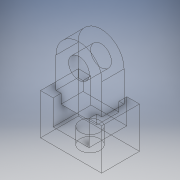
# Autodesk Inventor part: connectiong-rod-star-side
Saved by Autodesk Inventor 2018 (Build 220112000, 112)
## iProperties
Created: 2025-07-17
Part Number: connectiong-rod-star-side
Material: Generic
Document SubType Name: Modeling
Designer: neo
Density: 1 g/cm^3
Appearance: Default
Author: neo
Autodesk Inventor part; units mm, degrees
ref_plane "YZ Plane" through (0, 0, 0) normal (1, 0, 0) x (0, 1, 0)
ref_plane "XZ Plane" through (0, 0, 0) normal (0, 1, 0) x (-1, 0, 0)
ref_plane "XY Plane" through (0, 0, 0) normal (0, 0, 1) x (1, 0, 0)
sketch "Sketch1" plane through (0, 0, 0) normal (0, 1, 0) x (-1, 0, 0)
  circle A0 centre (0, 0) radius 1.65
  arc A1 (3.65, 0) -> (-3.65, 0) centre (0, 0) ccw
  line L0 (-3.65, 0) -> (-3.65, -11.35)
  line L1 (-3.65, -11.35) -> (3.65, -11.35)
  line L2 (3.65, -11.35) -> (3.65, 0)
  line L3 (0, 0) -> (0, -26.2529)
  line L4 (2.85, -11.35) -> (-2.85, -11.35)
  line L5 (-2.85, -9.35) -> (-2.85, -6.35)
  line L6 (-2.85, -6.35) -> (2.85, -6.35)
  line L7 (2.85, -6.35) -> (2.85, -9.35)
  line L8 (2.85, -9.35) -> (-2.85, -9.35)
  dimension "d0" = 3.3
  dimension "d1" = 2
  dimension "d2" = 15
  dimension "d3" = 5.7
  dimension "d4" = 5
  dimension "d5" = 2
  dimension "d13" = 3.65
  dimension "d14" = 7.3
  dimension "d15" = 0.8
  constraints: 18 end point, 3 parallel, 2 centre point, 2 coincident, 2 perpendicular, 2 point on circle, 2 tangent, 1 horizontal, 1 point on line, 1 vertical, 1 other
  measures "d0" diameter of A0
  measures "d1" radial gap between concentric circles of A1 A0
  measures "d3" distance between parallel lines of L5 L7
  measures "d4" distance of L6.end L4.start
  measures "d5" distance between parallel lines of L1 L8
  measures "d13" radius of A1
  measures "d14" distance between parallel lines of L0 L2
  measures "d15" distance between parallel lines of L7 L2
extrude "Extrusion1" add sketch "Sketch1" along normal mid plane 3.5
sketch "Sketch3" plane through (0, 0, 0) normal (0, 1, 0) x (-1, 0, 0)
  line L0 (-2.85, -6.35) -> (2.85, -6.35) construction
  line L1 (2.85, -6.35) -> (2.85, -9.35) construction
  line L2 (2.85, -9.35) -> (-2.85, -9.35) construction
  line L3 (-2.85, -9.35) -> (-2.85, -6.35) construction
  circle A0 centre (0, 0) radius 1.65 construction
  arc A1 (3.65, 0) -> (-3.65, 0) centre (0, 0) ccw construction
  line L4 (-3.65, 0) -> (-3.65, -11.35) projected
  line L5 (-3.65, -11.35) -> (3.65, -11.35) projected
  line L6 (3.65, -11.35) -> (3.65, 0) projected
  line L7 (3.65, -11.35) -> (-3.65, -11.35)
  line L8 (-3.65, -11.35) -> (-3.65, -8.85)
  line L9 (-3.65, -8.85) -> (3.65, -8.85)
  line L10 (3.65, -8.85) -> (3.65, -11.35)
  line L11 (4.85, -4.85) -> (2.85, -4.85)
  line L12 (2.85, -4.85) -> (2.85, -11.35)
  line L13 (2.85, -11.35) -> (4.85, -11.35)
  line L14 (4.85, -11.35) -> (4.85, -4.85)
  line L15 (-2.85, -4.85) -> (-4.85, -4.85)
  line L16 (-4.85, -4.85) -> (-4.85, -11.35)
  line L17 (-4.85, -11.35) -> (-2.85, -11.35)
  line L18 (-2.85, -11.35) -> (-2.85, -4.85)
  line L19 (-2.85, -9.35) -> (-2.85, -6.35) projected
  line L20 (2.85, -6.35) -> (2.85, -9.35) projected
  dimension "d16" = 2
  dimension "d17" = 1.5
  constraints: 24 end point, 6 parallel, 4 point on line, 3 collinear, 3 horizontal, 3 perpendicular
  measures "d16" distance between parallel lines of L12 L14
  measures "d17" distance between parallel lines of L11 L0
extrude "Extrusion2" add sketch "Sketch3" along normal mid plane 6
sketch "Sketch5" plane through (4.85, 3, -11.35) normal (0, 0, -1) x (-1, 0, 0)
  circle A0 centre (4.85, -3) radius 1.6
  dimension "d18" = 3.2
  constraints: 1 centre point, 1 coincident
  measures "d18" diameter of A0
extrude "Extrusion4" cut sketch "Sketch5" against normal up to surface (2.5 mm away)
body "Solid1"
